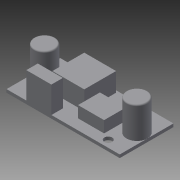
# Autodesk Inventor part: DC menic
Saved by Autodesk Inventor 2016 (Build 200138000, 138)
## iProperties
Created: 2015-11-16
Part Number: DC menic
Material: Generic
Document SubType Name: Modeling
Designer: Jufo
Density: 1 g/cm^3
Appearance: Default
Author: Jufo
Autodesk Inventor part; units mm, degrees
ref_plane "YZ Plane" through (0, 0, 0) normal (1, 0, 0) x (0, 1, 0)
ref_plane "XZ Plane" through (0, 0, 0) normal (0, 1, 0) x (-1, 0, 0)
ref_plane "XY Plane" through (0, 0, 0) normal (0, 0, 1) x (1, 0, 0)
sketch "Sketch1" plane through (0, 0, 0) normal (0, 1, 0) x (-1, 0, 0)
  line L0 (7.7899, 9.4408) -> (-35.6101, 9.4408)
  line L1 (-35.6101, 9.4408) -> (-35.6101, -11.1592)
  line L2 (-35.6101, -11.1592) -> (7.7899, -11.1592)
  line L3 (7.7899, -11.1592) -> (7.7899, 9.4408)
  point P0 (0, 0)
  dimension "d0" = 43.4
  dimension "d1" = 20.6
  constraints: 8 end point, 2 parallel, 1 horizontal, 1 perpendicular
  measures "d0" distance of L2.end L1.end
  measures "d1" distance of L1.end L0.end
extrude "Extrusion1" add sketch "Sketch1" along normal blind 1.2
sketch "Sketch2" plane through (0, 1.2, 0) normal (0, 1, 0) x (1, 0, 0)
  circle A0 centre (31.6101, 1.1592) radius 4
  line L0 (35.6101, 11.1592) -> (-7.7899, 11.1592) projected
  circle A1 centre (-3.7899, 1.1592) radius 4
  line L1 (-7.7899, 11.1592) -> (-7.7899, -9.4408) projected
  line L2 (35.6101, -9.4408) -> (35.6101, 11.1592) projected
  point P0 (0, 0)
  dimension "d4" = 8
  dimension "d5" = 10
  dimension "d6" = 8
  dimension "d7" = 4
  dimension "d8" = 4
  constraints: 2 centre point
  measures "d4" diameter of A0
  measures "d5" distance from line of L0 A0.centre
  measures "d6" diameter of A1
  measures "d7" distance from line of A1.centre L1
  measures "d8" distance from line of L2 A0.centre
extrude "Extrusion2" add sketch "Sketch2" along normal blind 12
fillet "Fillet1" radius 0.5 2 edges at (27.6101, 13.2, -1.1592) (-7.7899, 13.2, -1.1592)
sketch "Sketch3" plane through (0, 1.2, 0) normal (0, 1, 0) x (1, 0, 0)
  line L0 (9.4101, -5.0408) -> (-0.1899, -5.0408)
  line L1 (-0.1899, -5.0408) -> (-0.1899, -9.4408)
  line L2 (-0.1899, -9.4408) -> (9.4101, -9.4408)
  line L3 (9.4101, -9.4408) -> (9.4101, -5.0408)
  line L4 (-7.7899, -9.4408) -> (35.6101, -9.4408) projected
  line L5 (-7.7899, 1.1592) -> (-7.7899, -9.4408) projected
  point P0 (0, 0)
  dimension "d12" = 9.6
  dimension "d13" = 4.4
  dimension "d14" = 0
  dimension "d15" = 7.6
  constraints: 8 end point, 2 parallel, 1 horizontal, 1 perpendicular
  measures "d12" distance of L2.end L1.end
  measures "d13" distance of L1.end L0.end
  measures "d14" distance between parallel lines of L4 L2
  measures "d15" distance between parallel lines of L5 L1
extrude "Extrusion3" add sketch "Sketch3" along normal blind 10.1
sketch "Sketch4" plane through (0, 1.2, 0) normal (0, 1, 0) x (1, 0, 0)
  circle A0 centre (28.5101, -6.7408) radius 1.5
  line L0 (35.6101, -9.4408) -> (35.6101, 1.1592) projected
  line L1 (-7.7899, -9.4408) -> (35.6101, -9.4408) projected
  circle A1 centre (-1.2899, 8.4592) radius 1.5
  line L2 (35.6101, 11.1592) -> (-7.7899, 11.1592) projected
  line L3 (-7.7899, 11.1592) -> (-7.7899, -9.4408) projected
  point P0 (0, 0)
  dimension "d18" = 3
  dimension "d19" = 7.1
  dimension "d20" = 2.7
  dimension "d21" = 3
  dimension "d22" = 2.7
  dimension "d23" = 6.5
  constraints: 2 centre point
  measures "d18" diameter of A0
  measures "d19" distance from line of L0 A0.centre
  measures "d20" distance from line of L1 A0.centre
  measures "d21" diameter of A1
  measures "d22" distance from line of L2 A1.centre
  measures "d23" distance from line of L3 A1.centre
extrude "Extrusion4" cut sketch "Sketch4" against normal blind 10.1
sketch "Sketch5" plane through (0, 1.2, 0) normal (0, 1, 0) x (1, 0, 0)
  line L0 (14.4101, -1.8408) -> (2.2101, -1.8408)
  line L1 (2.2101, -1.8408) -> (2.2101, 10.3592)
  line L2 (2.2101, 10.3592) -> (14.4101, 10.3592)
  line L3 (14.4101, 10.3592) -> (14.4101, -1.8408)
  line L4 (35.6101, 11.1592) -> (-7.7899, 11.1592) projected
  line L5 (-7.7899, 11.1592) -> (-7.7899, 1.1592) projected
  point P0 (0, 0)
  dimension "d26" = 12.2
  dimension "d27" = 12.2
  dimension "d28" = 0.8
  dimension "d29" = 10
  constraints: 8 end point, 2 parallel, 1 horizontal, 1 perpendicular
  measures "d26" distance of L0.end L1.end
  measures "d27" distance of L0.start L0.end
  measures "d28" distance between parallel lines of L4 L2
  measures "d29" distance between parallel lines of L5 L1
extrude "Extrusion5" add sketch "Sketch5" along normal blind 7.2
sketch "Sketch6" plane through (0, 1.2, 0) normal (0, 1, 0) x (1, 0, 0)
  line L0 (25.6101, 2.9592) -> (15.6101, 2.9592)
  line L1 (15.6101, 2.9592) -> (15.6101, -5.4408)
  line L2 (15.6101, -5.4408) -> (25.6101, -5.4408)
  line L3 (25.6101, -5.4408) -> (25.6101, 2.9592)
  line L4 (9.4101, -9.4408) -> (35.6101, -9.4408) projected
  line L5 (35.6101, -9.4408) -> (35.6101, 1.1592) projected
  point P0 (0, 0)
  dimension "d32" = 10
  dimension "d33" = 8.4
  dimension "d34" = 4
  dimension "d35" = 10
  constraints: 8 end point, 2 parallel, 1 horizontal, 1 perpendicular
  measures "d32" distance of L2.end L1.end
  measures "d33" distance of L1.end L0.end
  measures "d34" distance between parallel lines of L4 L2
  measures "d35" distance between parallel lines of L3 L5
extrude "Extrusion6" add sketch "Sketch6" along normal blind 4.4
body "Solid1"
